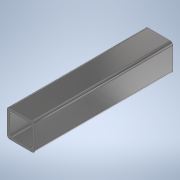
# Autodesk Inventor part: beam 20x20x2
Saved by Autodesk Inventor 2021 (Build 250183000, 183)
## iProperties
Created: 2024-04-08
Part Number: beam 20x20x2
Material: Steel
Document SubType Name: Modeling
Designer: Michal
Density: 7.85 g/cm^3
Appearance: Semi-Polished
Author: Michal
Autodesk Inventor part; units mm, degrees
ref_plane "YZ Plane" through (0, 0, 0) normal (1, 0, 0) x (0, 1, 0)
ref_plane "XZ Plane" through (0, 0, 0) normal (0, 1, 0) x (-1, 0, 0)
ref_plane "XY Plane" through (0, 0, 0) normal (0, 0, 1) x (1, 0, 0)
sketch "Sketch1" plane through (0, 0, 0) normal (0, 1, 0) x (-1, 0, 0)
  line L0 (-8, -10) -> (8, -10)
  line L1 (10, -8) -> (10, 8)
  line L2 (8, 10) -> (-8, 10)
  line L3 (-10, 8) -> (-10, -8)
  line L4 (-10, -10) -> (10, 10) construction
  line L5 (10, -10) -> (-10, 10) construction
  line L6 (-6, -8) -> (6, -8)
  line L7 (8, -6) -> (8, 6)
  line L8 (6, 8) -> (-6, 8)
  line L9 (-8, 6) -> (-8, -6)
  line L10 (-8, -8) -> (8, 8) construction
  line L11 (8, -8) -> (-8, 8) construction
  arc A0 (10, 8) -> (8, 10) centre (8, 8) ccw
  arc A1 (8, 6) -> (6, 8) centre (6, 6) ccw
  arc A2 (8, -10) -> (10, -8) centre (8, -8) ccw
  arc A3 (6, -8) -> (8, -6) centre (6, -6) ccw
  arc A4 (-10, -8) -> (-8, -10) centre (-8, -8) ccw
  arc A5 (-8, -6) -> (-6, -8) centre (-6, -6) ccw
  arc A6 (-6, 8) -> (-8, 6) centre (-6, 6) ccw
  arc A7 (-8, 10) -> (-10, 8) centre (-8, 8) ccw
  point P0 (0, 0)
  dimension "width" = 20
  dimension "depth" = 20
  dimension "thickness" = 2
  dimension "d3" = 2
  constraints: 24 end point, 17 point on line, 16 point on circle, 16 tangent, 8 centre point, 7 equal radius, 4 midpoint, 4 parallel, 2 horizontal, 2 perpendicular
  measures "width" distance of L5.end L4.end
  measures "depth" distance of L4.end L5.start
  measures "thickness" distance between parallel lines of L7 L1
  measures "d3" radius of A0
extrude "Extrusion1" add sketch "Sketch1" along normal blind 100
equation "\"d3\" = thickness"
body "Solid1"
